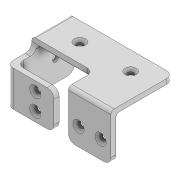
# Autodesk Inventor part: кронштейн
Saved by Autodesk Inventor 2021 (Build 250183000, 183)
## iProperties
Created: 2023-02-16
Part Number: кронштейн
Material: Типовые
Document SubType Name: Modeling
Designer: Tasya
Density: 1 g/cm^3
Appearance: По умолчанию
Author: Tasya
Autodesk Inventor part; units mm, degrees
ref_plane "YZ Plane" through (0, 0, 0) normal (1, 0, 0) x (0, 1, 0)
ref_plane "XZ Plane" through (0, 0, 0) normal (0, 1, 0) x (-1, 0, 0)
ref_plane "XY Plane" through (0, 0, 0) normal (0, 0, 1) x (1, 0, 0)
sketch "Эскиз1" plane through (0, 0, 0) normal (0, 1, 0) x (-1, 0, 0)
  line L0 (-29.25, 11) -> (29.25, 11)
  line L1 (29.25, 11) -> (29.25, -11)
  line L2 (29.25, -11) -> (-29.25, -11)
  line L3 (-29.25, -11) -> (-29.25, 11)
  line L4 (-29.25, 11) -> (29.25, -11) construction
  line L5 (29.25, 11) -> (-29.25, -11) construction
  line L6 (-29.25, 11) -> (-4.25, 11)
  line L7 (-4.25, 11) -> (-4.25, 23)
  line L8 (-4.25, 23) -> (-29.25, 23)
  line L9 (-29.25, 23) -> (-29.25, 11)
  point P0 (0, 0)
  dimension "d0" = 22
  dimension "d1" = 58.5
  dimension "d8" = 34
  dimension "d9" = 25
  constraints: 20 end point, 4 parallel, 2 midpoint, 2 perpendicular, 1 horizontal, 1 point on line
  measures "d0" distance of L2.end L0.start
  measures "d1" distance of L1.end L2.end
  measures "d8" distance between parallel lines of L2 L8
  measures "d9" distance of L7.end L8.end
extrude "Выдавливание1" add sketch "Эскиз1" along normal blind 3
sketch "Эскиз2" plane through (-29.25, 0, -11) normal (-1, 0, 0) x (0, 0, 1)
  line L0 (0, 0) -> (22, 0) projected
  line L1 (22, 0) -> (22, 3) projected
  line L2 (0, 3) -> (22, 3) projected
  line L3 (0, 0) -> (0, 3) projected
  line L4 (0, 3) -> (22, 3) projected
  line L5 (22, 3) -> (0, 3)
  line L6 (0, 3) -> (0, -25)
  line L7 (0, -25) -> (22, -25)
  line L8 (22, -25) -> (22, 3)
  line L9 (22, -25) -> (22, -3.9)
  line L10 (22, -3.9) -> (34, -3.9)
  line L11 (34, -3.9) -> (34, -25)
  line L12 (34, -25) -> (22, -25)
  point P0 (11, 0)
  point P1 (22, 0)
  point P2 (22, 3)
  dimension "d4" = 28
  dimension "d7" = 22
  dimension "d13" = 34
  dimension "d14" = 21.1
  constraints: 16 end point, 3 equal length, 3 perpendicular, 2 point on line, 1 horizontal
  measures "d4" distance of L2.start L6.end
  measures "d7" distance of L6.end L7.end
  measures "d13" distance between parallel lines of L11 L6
  measures "d14" distance of L10.end L11.end
extrude "Выдавливание2" add sketch "Эскиз2" along normal blind 3
sketch "Эскиз3" plane through (4.25, 0, 23) normal (0, 0, 1) x (1, 0, 0)
  line L0 (0, 0) -> (25, 0) projected
  line L1 (25, 0) -> (25, 3) projected
  line L2 (0, 3) -> (25, 3) projected
  line L3 (0, 0) -> (0, 3) projected
  line L4 (25, 0) -> (25, 3) projected
  line L5 (0, 0) -> (0, 3) projected
  line L6 (25, 3) -> (0, 3)
  line L7 (0, 3) -> (0, -25)
  line L8 (0, -25) -> (25, -25)
  line L9 (25, -25) -> (25, 3)
  point P0 (-4.25, 0)
  dimension "d10" = 28
  constraints: 8 end point, 2 parallel, 2 perpendicular
  measures "d10" distance between parallel lines of L2 L8
extrude "Выдавливание3" add sketch "Эскиз3" along normal blind 3
sketch "Эскиз4" plane through (-29.25, -25, 23) normal (0, 0, 1) x (1, 0, 0)
  line L0 (0, 0) -> (0, 21.1) projected
  line L1 (0, 21.1) -> (-3, 21.1) projected
  line L2 (-3, 0) -> (-3, 21.1) projected
  line L3 (0, 0) -> (-3, 0) projected
  line L4 (-3, 0) -> (-3, 21.1)
  line L5 (-3, 21.1) -> (25, 21.1)
  line L6 (25, 21.1) -> (25, 0)
  line L7 (25, 0) -> (-3, 0)
  point P0 (29.25, 25)
  dimension "d15" = 28
  constraints: 8 end point, 2 parallel, 1 perpendicular, 1 vertical
  measures "d15" distance of L6.end L2.start
extrude "Выдавливание4" add sketch "Эскиз4" along normal blind 3
fillet "Сопряжение1" radius 2 4 edges at (-29.25, 0, 0) (-32.25, 3, 0) (16.75, 3, 26) (16.75, 0, 23)
fillet "Сопряжение1" radius 4 10 edges at (-32.25, -14.45, 26) (-29.25, -14.45, 23) (-4.25, -3.9, 24.5) (-4.25, -25, 24.5) (-30.75, -3.9, 11) (4.25, 1.5, 11) (4.25, -25, 24.5) (29.25, -25, 24.5) (-30.75, -25, -11) (29.25, 1.5, -11)
sketch "Эскиз5" plane through (4.25, 0, 26) normal (0, 0, 1) x (1, 0, 0)
  circle A0 centre (6, -14.45) radius 1.8
  circle A1 centre (19, -14.45) radius 1.8
  arc A2 (21, -25) -> (25, -21) centre (21, -21) ccw projected
  line L0 (25, -21) -> (25, 1) projected
  line L1 (0, 1) -> (25, 1) projected
  line L2 (0, 1) -> (0, -21) projected
  arc A3 (0, -21) -> (4, -25) centre (4, -21) ccw projected
  line L3 (4, -25) -> (21, -25) projected
  line L4 (4, -25) -> (21, -25) construction
  line L5 (12.5, -25) -> (12.5, 1) construction
  line L6 (6, -14.45) -> (19, -14.45) construction
  line L7 (0, 0) -> (25, 0) construction
  arc A4 (-12.5, -25) -> (-8.5, -21) centre (-12.5, -21) ccw projected
  line L8 (-8.5, -21) -> (-8.5, -7.9) projected
  arc A5 (-8.5, -7.9) -> (-12.5, -3.9) centre (-12.5, -7.9) ccw projected
  line L9 (-12.5, -3.9) -> (-32.5, -3.9) projected
  line L10 (-32.5, -25) -> (-32.5, -3.9) projected
  line L11 (-32.5, -25) -> (-12.5, -25) projected
  line L12 (-36.5, -3.9) -> (-36.5, -25) projected
  circle A6 centre (-19.5, -19.45) radius 2.2361
  circle A7 centre (-19.5, -9.45) radius 2.6907
  line L13 (-19.5, -19.45) -> (-19.5, -9.45) construction
  line L14 (-19.5, -14.45) -> (-4.25, -14.45) construction
  point P0 (-4.25, 0)
  dimension "d21" = 3.6
  dimension "d22" = 3.6
  dimension "d23" = 13
  dimension "d33" = 13
  dimension "d34" = 10
  dimension "d35" = 21.1
  dimension "d36" = 10.55
  constraints: 8 end point, 4 centre point, 3 midpoint, 2 horizontal, 1 collinear, 1 symmetric about line, 1 vertical
  measures "d21" diameter of A0
  measures "d22" diameter of A1
  measures "d23" distance of L6.start L6.end
  measures "d33" distance between parallel lines of L10 L13
  measures "d34" distance of L13.start L13.end
  measures "d35" distance between parallel lines of L9 L11
  measures "d36" distance between parallel lines of L11 L14
hole "Отверстие1" at (10.25, -14.45, 26) at (23.25, -14.45, 26) at (-15.25, -9.45, 26) at (-15.25, -19.45, 26) direction (0, 0, -1) diameter 3.6 depth 5 countersink diameter 6.6 countersink angle 90 clearance for "с потайной головкой ГОСТ 12876-67" size "M3" standard "ГОСТ"
sketch "Эскиз6" plane through (-32.25, 0, -11) normal (-1, 0, 0) x (0, 0, 1)
  line L0 (32, 0) -> (4, 0) construction
  line L1 (22, 0) -> (0, 0) construction
  line L2 (0, 0) -> (0, -25) construction
  line L3 (0, -25) -> (22, -25) construction
  line L4 (22, -25) -> (22, 0) construction
  arc A0 (0, -21) -> (4, -25) centre (4, -21) ccw construction
  line L5 (4, -25) -> (33, -25) construction
  line L6 (33, -3.9) -> (33, -25) construction
  line L7 (26, -3.9) -> (33, -3.9) construction
  arc A1 (22, 0.1) -> (26, -3.9) centre (26, 0.1) ccw construction
  line L8 (22, 0.1) -> (22, 1) construction
  line L9 (0, 1) -> (22, 1) construction
  line L10 (0, 1) -> (0, -21) construction
  circle A2 centre (11, -12.5) radius 2.7933
  arc A3 (22, 0.1) -> (26, -3.9) centre (26, 0.1) ccw construction
  line L11 (22, 0.1) -> (0, -25) construction
  line L12 (0, 0) -> (0, -2) construction
  line L13 (22, -25) -> (0, 0) construction
  point P0 (11, 0)
  constraints: 12 end point, 4 collinear, 2 parallel, 1 centre point, 1 coincident, 1 midpoint, 1 perpendicular, 1 point on line
hole "Отверстие2" at (-32.25, -12.5, 0) direction (1, 0, 0) diameter 3.6 depth 6 countersink diameter 6.6 countersink angle 90 clearance for "с потайной головкой ГОСТ 12876-67" size "M3" standard "ГОСТ"
sketch "Эскиз7" plane through (0, 3, 0) normal (0, 1, 0) x (1, 0, 0)
  arc A0 (29.25, 7) -> (25.25, 11) centre (25.25, 7) ccw construction
  line L0 (25.25, 11) -> (-30.25, 11) construction
  line L1 (-30.25, -11) -> (-30.25, 11) construction
  line L2 (0.25, -11) -> (-30.25, -11) construction
  arc A1 (4.25, -15) -> (0.25, -11) centre (0.25, -15) ccw construction
  line L3 (4.25, -15) -> (4.25, -24) construction
  line L4 (29.25, -24) -> (4.25, -24) construction
  line L5 (29.25, 7) -> (29.25, -24) construction
  line L6 (29.25, -11) -> (29.25, 11) construction
  line L7 (29.25, 11) -> (-29.25, 11) construction
  line L8 (29.25, 7) -> (29.25, -24) construction
  line L9 (-29.2407, 0) -> (29.25, 0) construction
  line L10 (29.25, -21) -> (29.25, 7) construction
  line L11 (-29.25, -11.5956) -> (-29.25, 11) construction
  line L12 (-29.25, -11) -> (-29.25, 11) construction
  line L13 (-29.25, -11) -> (29.25, -11) construction
  circle A2 centre (-15, 0) radius 3.1623 construction
  circle A3 centre (15, 0) radius 5 construction
  line L14 (0, 0) -> (0, 6.5971) construction
  point P0 (-32.25, -11)
  point P1 (-29.25, 0)
  dimension "d44" = 30
  constraints: 13 end point, 7 point on line, 2 centre point, 2 collinear, 2 perpendicular, 1 horizontal, 1 midpoint, 1 parallel, 1 symmetric about line, 1 vertical
  measures "d44" distance of A3.centre A2.centre
hole "Отверстие3" at (-15, 3, 0) at (15, 3, 0) direction (0, -1, 0) diameter 3.6 depth 6 countersink diameter 6.6 countersink angle 90 clearance for "с потайной головкой ГОСТ 12876-67" size "M3" standard "ГОСТ"
equation "\"d36\" = 0.5 * d35"
